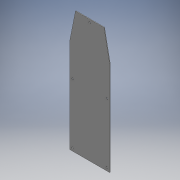
# Autodesk Inventor part: cover2
Saved by Autodesk Inventor 2016 (Build 200138000, 138)
## iProperties
Created: 2016-10-12
Part Number: cover2
Material: Generic
Document SubType Name: Modeling
Designer: Jakub
Density: 1 g/cm^3
Appearance: Default
Author: Jakub
Autodesk Inventor part; units mm, degrees
ref_plane "YZ Plane" through (0, 0, 0) normal (1, 0, 0) x (0, 1, 0)
ref_plane "XZ Plane" through (0, 0, 0) normal (0, 1, 0) x (-1, 0, 0)
ref_plane "XY Plane" through (0, 0, 0) normal (0, 0, 1) x (1, 0, 0)
sketch "Sketch1" plane through (0, 0, 0) normal (0, 1, 0) x (-1, 0, 0)
  line L0 (35, 107.75) -> (-35, 107.75)
  line L1 (-35, 107.75) -> (-35, -107.75)
  line L2 (-35, -107.75) -> (35, -107.75)
  line L3 (35, -107.75) -> (35, 107.75)
  line L4 (35, 107.75) -> (-35, -107.75) construction
  line L5 (-35, 107.75) -> (35, -107.75) construction
  circle A0 centre (30, -102.75) radius 1.5
  circle A1 centre (-30, -102.75) radius 1.5
  point P0 (0, 0)
  dimension "d0" = 70
  dimension "d1" = 215.5
  dimension "d2" = 3
  dimension "d3" = 3
  dimension "d4" = 5
  dimension "d5" = 5
  dimension "d6" = 5
  dimension "d7" = 5
  constraints: 12 end point, 2 centre point, 2 midpoint, 2 parallel, 1 horizontal, 1 perpendicular
  measures "d0" distance of L2.end L1.end
  measures "d1" distance of L1.end L0.end
  measures "d2" diameter of A0
  measures "d3" diameter of A1
  measures "d4" distance from line of L3 A0.centre
  measures "d5" distance from line of L2 A0.centre
  measures "d6" distance from line of L2 A1.centre
  measures "d7" distance from line of L1 A1.centre
extrude "Extrusion1" add sketch "Sketch1" along normal blind 1
sketch "Sketch2" plane through (0, 1, 0) normal (0, 1, 0) x (1, 0, 0)
  line L0 (-35, -107.75) -> (35, -107.75) projected
  line L1 (-35, -107.75) -> (-25, -107.75)
  line L2 (-25, -107.75) -> (-25, -57.75)
  line L3 (-25, -57.75) -> (-35, -57.75)
  line L4 (-35, -57.75) -> (-35, -107.75)
  line L5 (35, -107.75) -> (25, -107.75)
  line L6 (25, -107.75) -> (25, -57.75)
  line L7 (25, -57.75) -> (35, -57.75)
  line L8 (35, -57.75) -> (35, -107.75)
  line L9 (-25, -107.75) -> (-35, -57.75)
  line L10 (25, -107.75) -> (35, -57.75)
  point P0 (0, 0)
  dimension "d10" = 10
  dimension "d11" = 50
  dimension "d12" = 10
  dimension "d13" = 50
  constraints: 20 end point, 4 parallel, 2 horizontal, 2 perpendicular
  measures "d10" distance of L3.end L2.end
  measures "d11" distance of L2.end L1.end
  measures "d12" distance of L6.end L7.end
  measures "d13" distance of L5.end L6.end
extrude "Extrusion2" cut sketch "Sketch2" against normal up to next contours L4 L9 L0 | L10 L8 L0
sketch "Sketch3" plane through (0, 1, 0) normal (0, 1, 0) x (1, 0, 0)
  circle A0 centre (-30, -2.25) radius 1.5
  circle A1 centre (30, -2.25) radius 1.5
  line L0 (-25, -107.75) -> (25, -107.75) projected
  line L1 (-35, 107.75) -> (-35, -57.75) projected
  line L2 (35, -57.75) -> (35, 107.75) projected
  circle A2 centre (0, -102.75) radius 1.5
  point P0 (0, 0)
  dimension "d16" = 3
  dimension "d17" = 3
  dimension "d18" = 105.5
  dimension "d19" = 105.5
  dimension "d20" = 5
  dimension "d21" = 5
  dimension "d22" = 3
  dimension "d23" = 5
  constraints: 3 centre point
  measures "d16" diameter of A0
  measures "d17" diameter of A1
  measures "d18" distance from line of L0 A1.centre
  measures "d19" distance from line of L0 A0.centre
  measures "d20" distance from line of L1 A0.centre
  measures "d21" distance from line of L2 A1.centre
  measures "d22" diameter of A2
  measures "d23" distance from line of L0 A2.centre
extrude "Extrusion3" cut sketch "Sketch3" against normal up to next
body "Solid1"
